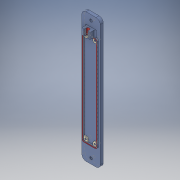
# Autodesk Inventor part: SH8_001.1-sunhub8-casing_bottom
Saved by Autodesk Inventor 2019 (Build 230136000, 136)
## iProperties
Created: 2019-02-22
Part Number: SH8_001.1-sunhub8-casing_bottom
Material: ABS Plastic
Document SubType Name: Modeling
Designer: Rene
Density: 1.06 g/cm^3
Appearance: Rubber - Blue
Author: Rene
Autodesk Inventor part; units mm, degrees
ref_plane "YZ Plane" through (0, 0, 0) normal (1, 0, 0) x (0, 1, 0)
ref_plane "XZ Plane" through (0, 0, 0) normal (0, 1, 0) x (-1, 0, 0)
ref_plane "XY Plane" through (0, 0, 0) normal (0, 0, 1) x (1, 0, 0)
sketch "Sketch1" plane through (0, 0, 0) normal (0, 0, 1) x (1, 0, 0)
  line L0 (-17.7, -125) -> (17.7, -125)
  line L1 (17.7, -125) -> (17.7, 125)
  line L2 (17.7, 125) -> (-17.7, 125)
  line L3 (-17.7, 125) -> (-17.7, -125)
  point P0 (0, 0)
  dimension "d0" = 250
  dimension "d1" = 125
  dimension "d2" = 35.4
  dimension "d3" = 17.7
  constraints: 8 end point, 2 parallel, 1 horizontal, 1 perpendicular
  measures "d0" distance of L2.end L0.start
  measures "d1" vertical distance of point (0, 0) L0.start
  measures "d2" distance of L0.start L0.end
  measures "d3" horizontal distance of point (0, 0) L0.start
extrude "Extrusion1" add sketch "Sketch1" along normal blind 6
fillet "Fillet1" radius 8 4 edges at (17.7, -125, 3) (-17.7, -125, 3) (17.7, 125, 3) (-17.7, 125, 3)
sketch "Sketch2" plane through (0, 0, 6) normal (0, 0, 1) x (1, 0, 0)
  line L0 (-14.7, 92.2) -> (14.7, 92.2)
  line L1 (14.7, 92.2) -> (14.7, -92.2)
  line L2 (14.7, -92.2) -> (-14.7, -92.2)
  line L3 (-14.7, -92.2) -> (-14.7, 92.2)
  point P0 (0, 0)
  dimension "d7" = 29.4
  dimension "d8" = 14.7
  dimension "d9" = 184.4
  dimension "d10" = 92.2
  constraints: 8 end point, 2 parallel, 1 horizontal, 1 perpendicular
  measures "d7" distance of L0.start L0.end
  measures "d8" horizontal distance of point (0, 0) L0.start
  measures "d9" distance of L1.end L0.end
  measures "d10" vertical distance of point (0, 0) L0.end
extrude "Extrusion2" add sketch "Sketch2" along normal blind 3
fillet "Fillet2" radius 4 4 edges at (-14.7, 92.2, 7.5) (14.7, 92.2, 7.5) (14.7, -92.2, 7.5) (-14.7, -92.2, 7.5)
sketch "Sketch3" plane through (0, 0, 9) normal (0, 0, 1) x (1, 0, 0)
  arc A0 (-14.7, -88.2) -> (-10.7, -92.2) centre (-10.7, -88.2) ccw projected
  line L0 (-10.7, -92.2) -> (10.7, -92.2) projected
  arc A1 (10.7, -92.2) -> (14.7, -88.2) centre (10.7, -88.2) ccw projected
  line L1 (14.7, -88.2) -> (14.7, 88.2) projected
  arc A2 (14.7, 88.2) -> (10.7, 92.2) centre (10.7, 88.2) ccw projected
  line L2 (10.7, 92.2) -> (-10.7, 92.2) projected
  arc A3 (-10.7, 92.2) -> (-14.7, 88.2) centre (-10.7, 88.2) ccw projected
  line L3 (-14.7, 88.2) -> (-14.7, -88.2) projected
  line L4 (-10.7, 90.2) -> (10.7, 90.2)
  arc A4 (12.7, 88.2) -> (10.7, 90.2) centre (10.7, 88.2) ccw
  line L5 (12.7, 88.2) -> (12.7, -88.2)
  arc A5 (10.7, -90.2) -> (12.7, -88.2) centre (10.7, -88.2) ccw
  line L6 (10.7, -90.2) -> (-10.7, -90.2)
  arc A6 (-12.7, -88.2) -> (-10.7, -90.2) centre (-10.7, -88.2) ccw
  line L7 (-12.7, -88.2) -> (-12.7, 88.2)
  arc A7 (-10.7, 90.2) -> (-12.7, 88.2) centre (-10.7, 88.2) ccw
  point P0 (0, 0)
  dimension "d14" = 2
  constraints: 8 end point, 8 point on circle, 4 centre point, 7 other
  measures "d14" distance between parallel lines of L4 L2
extrude "Extrusion3" cut sketch "Sketch3" against normal blind 3 contours L4 A4 L5 A5 L6 A6 L7 A7
sketch "Sketch4" plane through (0, 0, 0) normal (0, 0, -1) x (-1, 0, 0)
  line L0 (-9, 86.5) -> (9, 86.5) construction
  line L1 (9, 86.5) -> (9, -86.5) construction
  line L2 (9, -86.5) -> (-9, -86.5) construction
  line L3 (-9, -86.5) -> (-9, 86.5) construction
  point P0 (0, 0)
  dimension "d17" = 173
  dimension "d18" = 86.5
  dimension "d19" = 18
  dimension "d20" = 9
  constraints: 8 end point, 4 coincident, 2 parallel, 1 horizontal, 1 perpendicular
  measures "d17" distance of L2.end L0.start
  measures "d18" vertical distance of point (0, 0) L0.start
  measures "d19" distance of L0.start L0.end
  measures "d20" horizontal distance of point (0, 0) L0.start
hole "Hole1" at (-9, 86.5, 0) at (9, 86.5, 0) at (9, -86.5, 0) at (-9, -86.5, 0) direction (0, 0, 1) diameter 3.2 depth 20 tip angle 118 countersink diameter 6.5 countersink angle 90
sketch "Sketch5" plane through (0, 0, 6) normal (0, 0, 1) x (1, 0, 0)
  line L0 (-10.7, 90.2) -> (10.7, 90.2) projected
  line L1 (4.7, 90.2) -> (4.7, 82.2)
  line L2 (4.7, 82.2) -> (12.7, 82.2)
  line L3 (12.7, 88.2) -> (12.7, -88.2) projected
  arc A0 (12.7, 88.2) -> (10.7, 90.2) centre (10.7, 88.2) ccw projected
  circle A1 centre (9, 86.5) radius 1.6 projected
  point P0 (0, 0)
  dimension "d28" = 8
  dimension "d29" = 8
  constraints: 4 end point, 2 point on line, 1 perpendicular, 1 vertical
  measures "d28" distance of L1.start L1.end
  measures "d29" distance of L1.end L2.end
extrude "Extrusion5" add sketch "Sketch5" along normal blind 1.4
fillet "Fillet4" radius 4 1 edges at (4.7, 82.2, 6.7)
mirror "Mirror1" about plane through (0, 0, 0) normal (1, 0, 0) of "Extrusion5", "Fillet4"
mirror "Mirror2" about plane through (0, 0, 0) normal (0, 1, 0) of "Fillet4", "Extrusion5", "Mirror1"
sketch "Sketch6" plane through (0, 0, 6) normal (0, 0, 1) x (1, 0, 0)
  point P0 (0, 0)
  point P1 (0, 115)
  point P2 (0, -115)
  dimension "d36" = 230
  dimension "d37" = 115
  measures "d36" distance of point (0, -115) point (0, 115)
  measures "d37" distance of point (0, 0) point (0, 115)
hole "Hole2" at (0, 115, 6) at (0, -115, 6) direction (0, 0, -1) diameter 4.2 end through all
chamfer "Chamfer1" distance 0.5 angle 45 2 edges at (0, 117.1, 6) (0, -112.9, 6)
sketch "Sketch7" plane through (0, 0, 6) normal (0, 0, 1) x (1, 0, 0)
  line L0 (10.7, 92.2) -> (-10.7, 92.2) projected
  line L1 (-8, 104.2) -> (8, 104.2)
  line L2 (8, 104.2) -> (8, 92.2)
  line L3 (8, 92.2) -> (-8, 92.2)
  line L4 (-8, 92.2) -> (-8, 104.2)
  point P0 (0, 0)
  dimension "d48" = 16
  dimension "d49" = 8
  dimension "d50" = 12
  constraints: 8 end point, 2 parallel, 1 horizontal, 1 perpendicular, 1 point on line
  measures "d48" distance of L1.start L1.end
  measures "d49" horizontal distance of point (0, 0) L1.start
  measures "d50" distance of L1.end L2.end
extrude "Extrusion6" add sketch "Sketch7" along normal blind 10
sketch "Sketch8" plane through (0, 0, 16) normal (0, 0, 1) x (1, 0, 0)
  line L0 (8, 92.2) -> (-8, 92.2) projected
  line L1 (-3.25, 104.2) -> (3.25, 104.2)
  line L2 (3.25, 104.2) -> (3.25, 92.2)
  line L3 (3.25, 92.2) -> (-3.25, 92.2)
  line L4 (-3.25, 92.2) -> (-3.25, 104.2)
  line L5 (8, 104.2) -> (-8, 104.2) projected
  circle A0 centre (0, -115) radius 2.6 projected
  arc A1 (-9.7, 125) -> (-17.7, 117) centre (-9.7, 117) ccw projected
  line L6 (-17.7, 117) -> (-17.7, -117) projected
  arc A2 (-17.7, -117) -> (-9.7, -125) centre (-9.7, -117) ccw projected
  line L7 (-9.7, -125) -> (9.7, -125) projected
  arc A3 (9.7, -125) -> (17.7, -117) centre (9.7, -117) ccw projected
  line L8 (17.7, -117) -> (17.7, 117) projected
  arc A4 (17.7, 117) -> (9.7, 125) centre (9.7, 117) ccw projected
  line L9 (9.7, 125) -> (-9.7, 125) projected
  line L10 (-8, 92.2) -> (-8, 104.2) projected
  line L11 (-8, 104.2) -> (8, 104.2) projected
  line L12 (8, 104.2) -> (8, 92.2) projected
  line L13 (8, 92.2) -> (10.7, 92.2) projected
  arc A5 (14.7, 88.2) -> (10.7, 92.2) centre (10.7, 88.2) ccw projected
  line L14 (14.7, 88.2) -> (14.7, -88.2) projected
  arc A6 (10.7, -92.2) -> (14.7, -88.2) centre (10.7, -88.2) ccw projected
  line L15 (10.7, -92.2) -> (-10.7, -92.2) projected
  arc A7 (-14.7, -88.2) -> (-10.7, -92.2) centre (-10.7, -88.2) ccw projected
  line L16 (-14.7, -88.2) -> (-14.7, 88.2) projected
  arc A8 (-10.7, 92.2) -> (-14.7, 88.2) centre (-10.7, 88.2) ccw projected
  line L17 (-10.7, 92.2) -> (-8, 92.2) projected
  circle A9 centre (0, 115) radius 2.6 projected
  point P0 (0, 0)
  dimension "d53" = 6.5
  dimension "d54" = 3.25
  constraints: 8 end point, 2 parallel, 1 collinear, 1 horizontal, 1 perpendicular, 1 point on line
  measures "d53" distance between parallel lines of L2 L4
  measures "d54" horizontal distance of point (0, 0) L1.start
extrude "Extrusion7" cut sketch "Sketch8" against normal blind 7 contours L0 L4 L1 L2
fillet "Fillet5" radius 3.25 2 edges at (3.25, 98.2, 9) (-3.25, 98.2, 9)
fillet "Fillet6" radius 2.5 2 edges at (-8, 98.2, 6) (8, 98.2, 6)
fillet "Fillet7" radius 1 2 edges at (3.25, 98.2, 16) (-3.25, 98.2, 16)
equation "\"d1\" = 0.5 * d0"
equation "\"d3\" = 0.5 * d2"
equation "\"d8\" = 0.5 * d7"
equation "\"d10\" = 0.5 * d9"
equation "\"d18\" = 0.5 * d17"
equation "\"d20\" = 0.5 * d19"
equation "\"d29\" = d28"
equation "\"d37\" = 0.5 * d36"
equation "\"d49\" = 0.5 * d48"
equation "\"d54\" = 0.5 * d53"
body "Solid1"
